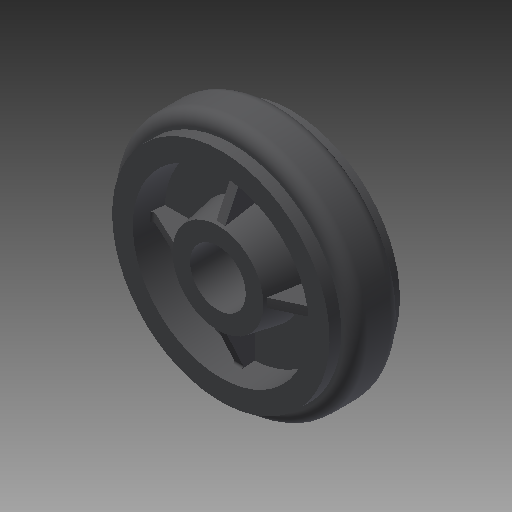
# Autodesk Inventor part: 3.00006.4411 1/2 (C)
Saved by Autodesk Inventor 2018 (Build 220112000, 112)
## iProperties
Category: PARTsolutions
Company: COLSONGROUP
Created: 2018-01-09
Part Number: 3.00006.4411 1/2 (C)
Catalog Web Link: www.cadenas.de
Description: Performa Rubber C-Wheels - Capacity up to 1700 lbs Each
Vendor: COLSONGROUP
Document SubType Name: Modeling
Designer: psAdmin
Manufacturer: COLSONGROUP
Mass: 320.529 g
Surface Area: 597.337 cm^2
Volume: 320.529 cm^3
Density: 1 g/cm^3
Material: Generic
Appearance: PSOLRGB-175-175-175
PSOL_IDENT_0: {$CADENAS_DATA\23d-libs\colsongroup\colson\wheels\performa_rubber\performa_rubber_core.prj},209 {VTY
PSOL_IDENT_1: P=3D},{NB=3.00006.4411 1/2 (C)},{LINA=3.00006.4411 1/2 (C)},{NN=Performa Rubber C},{DATE=12.06.2017
PSOL_IDENT_2: 06:51:29},{GEOMDATE=09.06.2017 06:04:28},{VERSION=},{LINEID=10},{LINESUBID=-1},{WBVAR=WT,SER,D,W,WB,
PSOL_IDENT_3: TG}  {NB=3.00006.4411 1/2 (C)},{LINA=3.00006.4411 1/2 (C)},{KT=DUMMY},{PN=3.00006.4411 1/2},{WH=Perf
PSOL_IDENT_4: orma Rubber},{WT=PRFG},{SER=3},{SERALG= '1','1 Series (Capacity up to 145 lbs)','2','2 Series (Capac
PSOL_IDENT_5: ity up to 325 lbs)','3','3 Series (Capacity up to 375 lbs)','4','4 Series (Capacity up to 500 lbs)','
PSOL_IDENT_6: 5','5 Series (Capacity up to 675 lbs)' },{D=6.00000000},{DALG=3,4,5,6},{DPN=06},{W=1.50000000},{WALG=
PSOL_IDENT_7: 1.5},{WTPN1=4},{WTPN2=4},{WTPN3=},{CAP=375},{CAPALG=375},{CAPPN=},{WB=1},{WBALG= '1','Delrin','9','R
PSOL_IDENT_8: oller','5','PPBB' },{WBPN=441},{TG=-},{TGALG= '-','N/A' },{TGPN=},{BB=0.50000000},{LBB=1.18750000},{
PSOL_IDENT_9: HUB=1.62500000},{SBB=0.37500000},{SBL=1.87500000},{WEIGHT=1.50000000},{CON=3},{D1=1.94},{D2=4.64},{B
PSOL_IDENT_10: ORE=1.19},{ANGS=6},{ANDT=3},{R1=0.25},{TT=0.31},{W1=0.25},{D3=3.76},{T=0.25},{ANGD=10},{ANGU=5},{T2=
PSOL_IDENT_11: 0.19},{T3=0.17},{CON2=2},{W2=1.25},{HUBR=1.625},{WR=1.5},{D4=5.44},{CPWB=0.8125},{CPWB2=0.8125},{TGC
PSOL_IDENT_12: P=0.9375},{SPCP=0.8975},{BORE2=1.5748},{BOREL=0.625}
NN: Performa Rubber C
NT: Wheels - Capacity up to 1700 lbs Each
NB: 3.00006.4411 1/2 (C)
NBSYN: $PN. (C)
LINA: 3.00006.4411 1/2 (C)
PN: 3.00006.4411 1/2
WH: Performa Rubber
WT: Flat Gray Thread
SER: 3 Series (Capacity up to 375 lbs)
D: 6
W: 1 1/2
WB: Delrin
TG: N/A
BB: 1/2
LBB: 1 3/16
HUB: 1 5/8
SBB: 3/8
SBL: 1 7/8
WEIGHT: 1 1/2
SUPPLIER: COLSONGROUP
ARTICLENO: 3.00006.4411 1/2 (C)
BOMINFO: 3.00006.4411 1/2 (C)
CREATOR: CADENAS GmbH
Title: 3.00006.4411 1/2 (C)
Author: Cadenas PARTsolutions
Comments: Wheels - Capacity up to 1700 lbs Each
Autodesk Inventor part; units mm, degrees
sketch "Sketch_1" plane through (0, 0, 0) normal (1, 0, 0) x (0, 1, 0)
  line L0 (0, -20.6375) -> (0, 20.6375)
  line L1 (0, 20.6375) -> (24.638, 20.6375)
  line L2 (24.638, 20.6375) -> (27.7171, 3.175)
  line L3 (27.7171, 3.175) -> (46.3631, 3.175)
  line L4 (46.3631, 3.175) -> (47.752, 19.05)
  line L5 (47.752, 19.05) -> (58.928, 19.05)
  line L6 (58.928, 19.05) -> (58.928, 12.7)
  line L7 (58.928, 12.7) -> (60.452, 12.7)
  arc A0 (66.802, 6.35) -> (60.452, 12.7) centre (60.452, 6.35) ccw
  line L8 (66.802, 6.35) -> (66.802, -6.35)
  arc A1 (60.452, -12.7) -> (66.802, -6.35) centre (60.452, -6.35) ccw
  line L9 (60.452, -12.7) -> (58.928, -12.7)
  line L10 (58.928, -12.7) -> (58.928, -19.05)
  line L11 (58.928, -19.05) -> (47.752, -19.05)
  line L12 (47.752, -19.05) -> (46.3631, -3.175)
  line L13 (46.3631, -3.175) -> (27.7171, -3.175)
  line L14 (27.7171, -3.175) -> (24.638, -20.6375)
  line L15 (24.638, -20.6375) -> (0, -20.6375)
  line L16 (0, -20.6375) -> (0, 20.6375)
  constraints: 34 end point, 4 point on circle, 2 centre point
revolve "Revolution1" add sketch "Sketch_1" angle 360 about axis through (0, 0, -20.6375) along (0, 0, -1)
sketch "Sketch_5" plane through (0, 0, 0) normal (0, 0, 1) x (1, 0, 0)
  arc A0 (-57.699, 2.413) -> (-57.699, -2.413) centre (0, 0) ccw
  line L0 (-57.699, -2.413) -> (-14.9191, -2.413)
  arc A1 (-14.9191, -2.413) -> (-2.413, -14.9191) centre (0, 0) ccw
  line L1 (-2.413, -14.9191) -> (-2.413, -57.699)
  arc A2 (-2.413, -57.699) -> (2.413, -57.699) centre (0, 0) ccw
  line L2 (2.413, -57.699) -> (2.413, -14.9191)
  arc A3 (2.413, -14.9191) -> (14.9191, -2.413) centre (0, 0) ccw
  line L3 (14.9191, -2.413) -> (57.699, -2.413)
  arc A4 (57.699, -2.413) -> (57.699, 2.413) centre (0, 0) ccw
  line L4 (57.699, 2.413) -> (14.9191, 2.413)
  arc A5 (14.9191, 2.413) -> (2.413, 14.9191) centre (0, 0) ccw
  line L5 (2.413, 14.9191) -> (2.413, 57.699)
  arc A6 (2.413, 57.699) -> (-2.413, 57.699) centre (0, 0) ccw
  line L6 (-2.413, 57.699) -> (-2.413, 14.9191)
  arc A7 (-2.413, 14.9191) -> (-14.9191, 2.413) centre (0, 0) ccw
  line L7 (-14.9191, 2.413) -> (-57.699, 2.413)
  constraints: 16 end point, 16 point on circle, 8 centre point
extrude "Extrusion1" add sketch "Sketch_5" along normal blind 19.05
sketch "Sketch_7" plane through (0, 0, 0) normal (0, 0, 1) x (1, 0, 0)
  arc A0 (-42.5056, -39.0931) -> (-39.0931, -42.5056) centre (0, 0) ccw
  line L0 (-39.0931, -42.5056) -> (-8.8432, -12.2557)
  arc A1 (-8.8432, -12.2557) -> (8.8432, -12.2557) centre (0, 0) ccw
  line L1 (8.8432, -12.2557) -> (39.0931, -42.5056)
  arc A2 (39.0931, -42.5056) -> (42.5056, -39.0931) centre (0, 0) ccw
  line L2 (42.5056, -39.0931) -> (12.2557, -8.8432)
  arc A3 (12.2557, -8.8432) -> (12.2557, 8.8432) centre (0, 0) ccw
  line L3 (12.2557, 8.8432) -> (42.5056, 39.0931)
  arc A4 (42.5056, 39.0931) -> (39.0931, 42.5056) centre (0, 0) ccw
  line L4 (39.0931, 42.5056) -> (8.8432, 12.2557)
  arc A5 (8.8432, 12.2557) -> (-8.8432, 12.2557) centre (0, 0) ccw
  line L5 (-8.8432, 12.2557) -> (-39.0931, 42.5056)
  arc A6 (-39.0931, 42.5056) -> (-42.5056, 39.0931) centre (0, 0) ccw
  line L6 (-42.5056, 39.0931) -> (-12.2557, 8.8432)
  arc A7 (-12.2557, 8.8432) -> (-12.2557, -8.8432) centre (0, 0) ccw
  line L7 (-12.2557, -8.8432) -> (-42.5056, -39.0931)
  constraints: 16 end point, 16 point on circle, 8 centre point
extrude "Extrusion2" add sketch "Sketch_7" against normal blind 19.05
sketch "Sketch_6" plane through (0, 0, 0) normal (1, 0, 0) x (0, 1, 0)
  line L0 (0, 20.6375) -> (0, 28.5115)
  line L1 (0, 28.5115) -> (47.752, 28.5115)
  line L2 (47.752, 28.5115) -> (47.752, 19.05)
  line L3 (47.752, 19.05) -> (47.015, 10.6265)
  arc A0 (45.2131, 9.5862) -> (47.015, 10.6265) centre (45.7499, 10.7372) ccw
  line L4 (45.2131, 9.5862) -> (24.9179, 19.05)
  line L5 (24.9179, 19.05) -> (24.638, 20.6375)
  line L6 (24.638, 20.6375) -> (0, 20.6375)
  line L7 (0, 20.6375) -> (0, 28.5115)
  constraints: 16 end point, 2 point on circle, 1 centre point
revolve "Revolution2" cut sketch "Sketch_6" angle 360 about axis through (0, 0, 20.6375) along (0, 0, -1)
sketch "Sketch_4" plane through (0, 0, 0) normal (1, 0, 0) x (0, 1, 0)
  line L0 (0, -28.5115) -> (0, -20.6375)
  line L1 (0, -20.6375) -> (24.638, -20.6375)
  line L2 (24.638, -20.6375) -> (24.9179, -19.05)
  line L3 (24.9179, -19.05) -> (45.2131, -9.5862)
  arc A0 (47.015, -10.6265) -> (45.2131, -9.5862) centre (45.7499, -10.7372) ccw
  line L4 (47.015, -10.6265) -> (47.752, -19.05)
  line L5 (47.752, -19.05) -> (47.752, -28.5115)
  line L6 (47.752, -28.5115) -> (0, -28.5115)
  line L7 (0, -28.5115) -> (0, -20.6375)
  constraints: 16 end point, 2 point on circle, 1 centre point
revolve "Revolution3" cut sketch "Sketch_4" angle 360 about axis through (0, 0, -28.5115) along (0, 0, -1)
sketch "Sketch_3_ALT_Drilling_1" plane through (0, 0, 0) normal (1, 0, 0) x (0, 1, 0)
  line L0 (0, -20.6375) -> (0, 20.6375)
  line L1 (0, 20.6375) -> (15.113, 20.6375)
  line L2 (15.113, 20.6375) -> (15.113, -20.6375)
  line L3 (15.113, -20.6375) -> (0, -20.6375)
  line L4 (0, -20.6375) -> (0, 20.6375)
  constraints: 10 end point
revolve "Revolution4" cut sketch "Sketch_3_ALT_Drilling_1" angle 360 about axis through (0, 0, -20.6375) along (0, 0, -1)
ref_plane "BB_1_XY" through (0, 6.35, -20.6375) normal (1, 0, 0) x (0, 0, -1)
ref_plane "BB_1_YZ" through (0, 6.35, -20.6375) normal (0, 0, -1) x (0, 1, 0)
ref_plane "BB_1_ZX" through (0, 6.35, -20.6375) normal (0, 1, 0) x (1, 0, 0)
ref_plane "BB_2_XY" through (0, -6.35, -20.6375) normal (1, 0, 0) x (0, 0, -1)
ref_plane "BB_2_YZ" through (0, -6.35, -20.6375) normal (0, 0, -1) x (0, 1, 0)
ref_plane "BB_2_ZX" through (0, -6.35, -20.6375) normal (0, 1, 0) x (1, 0, 0)
ref_plane "D_1_XY" through (0, 76.2, 0) normal (0, 0, 1) x (1, 0, 0)
ref_plane "D_1_YZ" through (0, 76.2, 0) normal (1, 0, 0) x (0, 1, 0)
ref_plane "D_1_ZX" through (0, 76.2, 0) normal (0, 1, 0) x (0, 0, 1)
ref_plane "D_2_XY" through (0, -76.2, 0) normal (0, 0, 1) x (1, 0, 0)
ref_plane "D_2_YZ" through (0, -76.2, 0) normal (1, 0, 0) x (0, 1, 0)
ref_plane "D_2_ZX" through (0, -76.2, 0) normal (0, 1, 0) x (0, 0, 1)
ref_plane "HUB_1_XY" through (0, -24.638, 20.6375) normal (1, 0, 0) x (0, 0, -1)
ref_plane "HUB_1_YZ" through (0, -24.638, 20.6375) normal (0, 0, -1) x (0, 1, 0)
ref_plane "HUB_1_ZX" through (0, -24.638, 20.6375) normal (0, 1, 0) x (1, 0, 0)
ref_plane "HUB_2_XY" through (0, -24.638, -20.6375) normal (1, 0, 0) x (0, 0, -1)
ref_plane "HUB_2_YZ" through (0, -24.638, -20.6375) normal (0, 0, -1) x (0, 1, 0)
ref_plane "HUB_2_ZX" through (0, -24.638, -20.6375) normal (0, 1, 0) x (1, 0, 0)
ref_plane "W_1_XY" through (0, 24.638, 19.05) normal (1, 0, 0) x (0, 0, -1)
ref_plane "W_1_YZ" through (0, 24.638, 19.05) normal (0, 0, -1) x (0, 1, 0)
ref_plane "W_1_ZX" through (0, 24.638, 19.05) normal (0, 1, 0) x (1, 0, 0)
ref_plane "W_2_XY" through (0, 24.638, -19.05) normal (1, 0, 0) x (0, 0, -1)
ref_plane "W_2_YZ" through (0, 24.638, -19.05) normal (0, 0, -1) x (0, 1, 0)
ref_plane "W_2_ZX" through (0, 24.638, -19.05) normal (0, 1, 0) x (1, 0, 0)
ref_plane "core_XY" through (0, 0, 0) normal (0, 0, 1) x (1, 0, 0)
ref_plane "core_YZ" through (0, 0, 0) normal (1, 0, 0) x (0, 1, 0)
ref_plane "core_ZX" through (0, 0, 0) normal (0, 1, 0) x (0, 0, 1)
ref_plane "core_to_bearing1_XY" through (0, 0, 20.6375) normal (0, 0, 1) x (1, 0, 0)
ref_plane "core_to_bearing1_YZ" through (0, 0, 20.6375) normal (1, 0, 0) x (0, 1, 0)
ref_plane "core_to_bearing1_ZX" through (0, 0, 20.6375) normal (0, 1, 0) x (0, 0, 1)
ref_plane "core_to_bearing2_XY" through (0, 0, -20.6375) normal (0, 0, 1) x (1, 0, 0)
ref_plane "core_to_bearing2_YZ" through (0, 0, -20.6375) normal (1, 0, 0) x (0, 1, 0)
ref_plane "core_to_bearing2_ZX" through (0, 0, -20.6375) normal (0, 1, 0) x (0, 0, 1)
ref_plane "core_to_tg1_XY" through (0, 0, 23.8125) normal (0, 0, 1) x (1, 0, 0)
ref_plane "core_to_tg1_YZ" through (0, 0, 23.8125) normal (1, 0, 0) x (0, 1, 0)
ref_plane "core_to_tg1_ZX" through (0, 0, 23.8125) normal (0, 1, 0) x (0, 0, 1)
ref_plane "core_to_tg2_XY" through (0, 0, -23.8125) normal (0, 0, 1) x (1, 0, 0)
ref_plane "core_to_tg2_YZ" through (0, 0, -23.8125) normal (1, 0, 0) x (0, 1, 0)
ref_plane "core_to_tg2_ZX" through (0, 0, -23.8125) normal (0, 1, 0) x (0, 0, 1)
ref_plane "to_spacer1_XY" through (0, 0, 22.7965) normal (0, 0, 1) x (1, 0, 0)
ref_plane "to_spacer1_YZ" through (0, 0, 22.7965) normal (1, 0, 0) x (0, 1, 0)
ref_plane "to_spacer1_ZX" through (0, 0, 22.7965) normal (0, 1, 0) x (0, 0, 1)
ref_plane "to_spacer2_XY" through (0, 0, -22.7965) normal (0, 0, 1) x (1, 0, 0)
ref_plane "to_spacer2_YZ" through (0, 0, -22.7965) normal (1, 0, 0) x (0, 1, 0)
ref_plane "to_spacer2_ZX" through (0, 0, -22.7965) normal (0, 1, 0) x (0, 0, 1)
ref_plane "to_washer1_XY" through (0, 0, 20.6375) normal (0, 0, 1) x (1, 0, 0)
ref_plane "to_washer1_YZ" through (0, 0, 20.6375) normal (1, 0, 0) x (0, 1, 0)
ref_plane "to_washer1_ZX" through (0, 0, 20.6375) normal (0, 1, 0) x (0, 0, 1)
ref_plane "to_washer2_XY" through (0, 0, -20.6375) normal (0, 0, 1) x (1, 0, 0)
ref_plane "to_washer2_YZ" through (0, 0, -20.6375) normal (1, 0, 0) x (0, 1, 0)
ref_plane "to_washer2_ZX" through (0, 0, -20.6375) normal (0, 1, 0) x (0, 0, 1)
body "Solid1"
